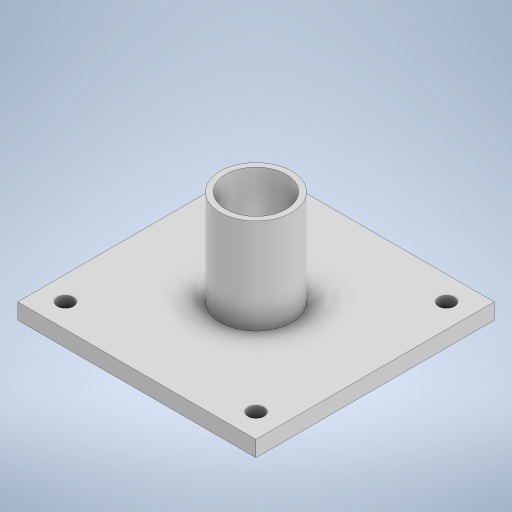
# Autodesk Inventor part: Motor_beam_connection
Saved by Autodesk Inventor 2024.2 (Build 282272000, 272)
## iProperties
Created: 2024-03-26
Part Number: Motor_beam_connection
Material: Generic
Document SubType Name: Modeling
Designer: feder
Density: 1 g/cm^3
Appearance: Default
Author: feder
Autodesk Inventor part; units mm, degrees
ref_plane "YZ Plane" through (0, 0, 0) normal (1, 0, 0) x (0, 1, 0)
ref_plane "XZ Plane" through (0, 0, 0) normal (0, 1, 0) x (-1, 0, 0)
ref_plane "XY Plane" through (0, 0, 0) normal (0, 0, 1) x (1, 0, 0)
sketch "Sketch1" plane through (0, 0, 0) normal (0, 1, 0) x (-1, 0, 0)
  line L0 (75, 75) -> (-75, 75)
  line L1 (-75, 75) -> (-75, -75)
  line L2 (-75, -75) -> (75, -75)
  line L3 (75, -75) -> (75, 75)
  line L4 (75, 75) -> (-75, -75) construction
  line L5 (-75, 75) -> (75, -75) construction
  point P0 (0, 0)
  dimension "d6" = 150
  dimension "d7" = 150
  constraints: 12 end point, 2 midpoint, 2 parallel, 1 horizontal, 1 perpendicular
  measures "d6" distance between parallel lines of L2 L0
  measures "d7" distance between parallel lines of L1 L3
extrude "Extrusion4" add sketch "Sketch1" along normal blind 10
sketch "Sketch4" plane through (0, 10, 0) normal (0, 1, 0) x (1, 0, 0)
  line L0 (75, 75) -> (-75, 75) projected
  line L1 (0, 0) -> (-75, 75) construction
  circle A0 centre (-60, 60) radius 5
  line L2 (-75, 75) -> (-75, -75) projected
  line L3 (0, 75) -> (0, -75) construction
  line L4 (-75, -75) -> (75, -75) projected
  line L5 (-75, 0) -> (75, 0) construction
  circle A1 centre (60, 60) radius 5
  circle A2 centre (-60, -60) radius 5
  circle A3 centre (60, -60) radius 5
  dimension "d10" = 10
  dimension "d11" = 15
  dimension "d12" = 15
  constraints: 6 end point, 4 centre point, 3 midpoint, 3 symmetric about line, 1 horizontal, 1 point on line, 3 other
  measures "d10" diameter of A0
  measures "d11" distance from line of L2 A0.centre
  measures "d12" distance from line of L0 A0.centre
extrude "Extrusion5" cut sketch "Sketch4" against normal through all
sketch "Sketch5" plane through (0, 10, 0) normal (0, 1, 0) x (1, 0, 0)
  circle A0 centre (0, 0) radius 22.5
  circle A1 centre (0, 0) radius 19.005
  dimension "d15" = 45
  dimension "d18" = 38.01
  constraints: 2 centre point, 2 coincident
  measures "d15" diameter of A0
  measures "d18" diameter of A1
extrude "Extrusion6" add sketch "Sketch5" along normal blind 60
body "Solid2"
